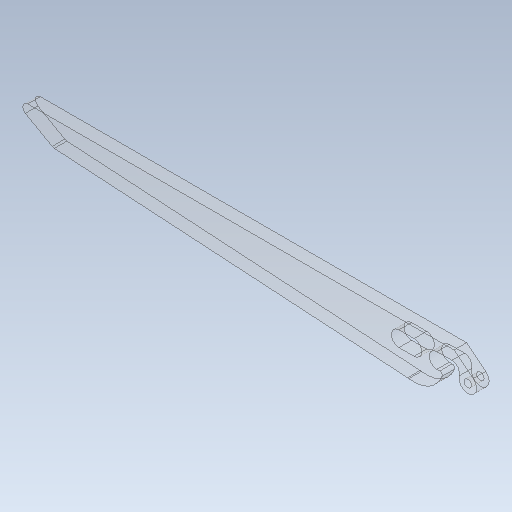
# Autodesk Inventor part: ウイング仮
Saved by Autodesk Inventor 2020 (Build 240168000, 168)
## iProperties
Created: 2019-06-21
Part Number: ウイング仮
Material: ポリカーボネート、クリア
Document SubType Name: Modeling
Designer: tanjihayato
Density: 1.2 g/cm^3
Appearance: ポリカーボネート - クリア
Mass: 13.8984 g
Surface Area: 68.0669 cm^2
Volume: 11.582 cm^3
Author: tanjihayato
Autodesk Inventor part; units mm, degrees
ref_plane "YZ Plane" through (0, 0, 0) normal (1, 0, 0) x (0, 1, 0)
ref_plane "XZ Plane" through (0, 0, 0) normal (0, 1, 0) x (-1, 0, 0)
ref_plane "XY Plane" through (0, 0, 0) normal (0, 0, 1) x (1, 0, 0)
sketch "スケッチ1" plane through (0, 0, 0) normal (0, 0, 1) x (1, 0, 0)
  arc A0 (-2.6047, -14.7721) -> (15, 0) centre (0, 0) ccw construction
  arc A1 (-2.0751, -11.7685) -> (11.5542, -3.05) centre (0, 0) ccw
  arc A2 (-2.0751, -11.7685) -> (-2.602, -11.7221) centre (-2.6047, -14.7721) ccw
  line L0 (0, 0) -> (-6, 0) construction
  line L1 (0, 3.05) -> (-6, 3.05)
  line L2 (-6, -3.05) -> (0, -3.05)
  arc A3 (0, -3.05) -> (0, 3.05) centre (0, 0) ccw
  arc A4 (-6, 3.05) -> (-6, -3.05) centre (-6, 0) ccw
  line L3 (15, 0) -> (9, 0) construction
  line L4 (15, 3.05) -> (9, 3.05)
  arc A5 (9, 3.05) -> (9, -3.05) centre (9, 0) ccw
  line L5 (-161, 7.05) -> (9, 7.05)
  line L6 (-161, 7.05) -> (-143.3628, -2.95)
  line L7 (-2.602, -11.7221) -> (-143.3628, -2.95)
  arc A6 (17.9444, -0.7957) -> (15, 3.05) centre (15, 0) ccw
  line L8 (9, -3.05) -> (11.5542, -3.05)
  line L9 (14.6866, -3.05) -> (14.3582, -3.05)
  circle A7 centre (21.3232, -1.7088) radius 1.5
  arc A8 (17.9444, -0.7957) -> (23.4882, 1.0412) centre (21.3232, -1.7088) ccw
  line L10 (9, 7.05) -> (15.8557, 7.05)
  line L11 (15.8557, 7.05) -> (23.4882, 1.0412)
  point P0 (-3, 0)
  point P1 (12, 0)
  dimension "d0" = 15
  dimension "d1" = 6.1
  dimension "d2" = 6
  dimension "d3" = 6.1
  dimension "d4" = 6
  dimension "d5" = 6.1
  dimension "d6" = 100
  dimension "d8" = 4
  dimension "d9" = 10
  dimension "d17" = 3
  dimension "d19" = 2
  dimension "d20" = 170
  constraints: 28 end point, 17 point on circle, 11 tangent, 9 centre point, 5 horizontal, 3 parallel, 2 coincident, 2 midpoint, 1 point on line
  measures "d0" radius of A0
  measures "d1" diameter of A2
  measures "d2" distance of L0.start L0.end
  measures "d3" diameter of A4
  measures "d4" distance of L3.start L3.end
  measures "d5" diameter of A5
  measures "d8" distance between parallel lines of L5 L1
  measures "d9" distance from line of L6.end L5
  measures "d17" diameter of A7
  measures "d19" radial gap between concentric circles of A8 A7
  measures "d20" distance of L5.start L5.end
extrude "押し出し1" add sketch "スケッチ1" along normal blind 5
fillet "フィレット1" radius 2 2 edges at (-161, 7.05, 2.5) (-143.3628, -2.95, 2.5)
fillet "フィレット3" radius 1 1 edges at (11.5542, -3.05, 2.5)
